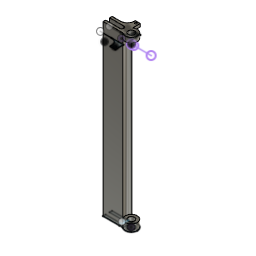
Aft_Flap (Autodesk Fusion 360 design; units mm, degrees)
Autodesk Fusion 360 part; units mm, degrees
note: some values were not read from the file. Set by a fixed rule: which sketch regions a step uses.
sketch "Sketch1" plane through (0, 0, 0) normal (0, 0, 1) x (1, 0, 0)
  circle A0 centre (0, 0) radius 3.2
  circle A1 centre (0, 0) radius 6
  line L0 (-7.5, -4.5) -> (-3.9686, -4.5)
  line L1 (-3.9686, -4.5) -> (-3.9686, 4.5)
  line L2 (-3.9686, 4.5) -> (-7.5, 4.5)
  line L3 (-7.5, 0) -> (-7.5, 0)
  line L4 (-7.5, 4.5) -> (-23.9686, 4.5)
  line L5 (-23.9686, 4.5) -> (-23.9686, 2)
  line L6 (-23.9686, 2) -> (-9.5, 2)
  line L7 (-7.5, 2) -> (-7.5, 4.5)
  line L8 (-7.5, -4.5) -> (-23.9686, -4.5)
  line L9 (-23.9686, -4.5) -> (-23.9686, -2)
  line L10 (-23.9686, -2) -> (-9.5, -2)
  line L11 (-7.5, -2) -> (-7.5, -4.5)
  arc A2 (-7.5, 0) -> (-9.5, 2) centre (-9.5, 0) ccw
  arc A3 (-9.5, -2) -> (-7.5, 0) centre (-9.5, 0) ccw
  dimension "d1" = 6.4
  dimension "d2" = 12
  dimension "d10" = 2
  dimension "d11" = 2
  dimension "d12" = 7.5
  dimension "d15" = 9
  dimension "d16" = 2
  dimension "d17" = 2
  dimension "d19" = 2.5
  dimension "d32" = 2.5
  dimension "d33" = 20
  dimension "d34" = 20
  constraint coincident A0.centre A1.centre
  constraint horizontal L2
  constraint coincident A1 L1.end
  constraint horizontal L4
  constraint vertical L5
  constraint horizontal L6
  constraint vertical L7
  constraint horizontal L8
  constraint vertical L9
  constraint horizontal L10
  constraint vertical L11
  constraint coincident L7.start L6
  constraint tangent L6 A2
  constraint coincident L0.start L3
  constraint coincident L11.start L10
  constraint tangent L10 A3
  constraint parallel L0 L8
  constraint coincident L1 L0.end
  constraint coincident L0.end L1.start
  constraint perpendicular L0 L1
  measures "d1" diameter of A0
  measures "d2" diameter of A1
  measures "d10" distance of A0.centre L10
  measures "d11" distance of A0.centre L6
  measures "d12" distance of A0.centre L11
  measures "d15" distance of L0.end L1.end
  measures "d16" radius of A2
  measures "d17" radius of A3
  measures "d19" distance of L4 L6
  measures "d32" distance of L8 L10
  measures "d33" distance of L1 L5
  measures "d34" distance of L1 L9
extrude "Extrude1" add sketch "Sketch1" along normal blind 7 contours A1 L1 | A1 L1 makes body 1
extrude "Extrude2" add sketch "Sketch1" along normal blind 5 from surface at 165 separate body contours A1 L1 | A1 L1 makes body 2
extrude "Extrude3" add sketch "Sketch1" along normal blind 170 contours A1 L0 L2 L4 L5 L6 L8 L9 L10 A2 A3 bodies 1 2
ref_plane "WorkPlane1" through (-7.8276, 0, 160) normal (0, 0, 1) x (1, 0, 0)
sketch "Sketch2" plane through (-9.7903, 0, 160) normal (0, 0, 1) x (1, 0, 0)
  line L0 (6.2903, -4.5) -> (1.2903, -4.5)
  line L1 (1.2903, -11.5) -> (1.2903, -12.5)
  line L2 (1.2903, -12.5) -> (6.2903, -12.5)
  line L3 (6.2903, -12.5) -> (6.2903, -4.5)
  circle A0 centre (3.7903, -10.5) radius 1
  line L4 (-5.7097, -4.5) -> (-16.9277, -4.5)
  arc A1 (1.2903, -11.5) -> (-5.7097, -4.5) centre (-5.7097, -11.5) ccw
  line L5 (1.2903, -4.5) -> (-5.7097, -4.5)
  line L6 (29.7903, 0) -> (12.2903, 0)
  line L7 (6.2903, 12.5) -> (6.2903, 4.5)
  line L8 (6.2903, 4.5) -> (1.2903, 4.5)
  circle A2 centre (3.7903, 10.5) radius 1
  arc A3 (-5.7097, 4.5) -> (1.2903, 11.5) centre (-5.7097, 11.5) ccw
  line L9 (1.2903, 4.5) -> (-5.7097, 4.5)
  line L10 (-5.7097, 4.5) -> (-16.9277, 4.5)
  line L11 (1.2903, 12.5) -> (6.2903, 12.5)
  line L12 (1.2903, 11.5) -> (1.2903, 12.5)
  point P0 (9.7903, 0)
  point P1 (9.7903, 0)
  dimension "d21" = 4.5
  dimension "d22" = 5
  dimension "d23" = 3.5
  dimension "d24" = 8
  dimension "d25" = 2
  dimension "d26" = 6
  dimension "d27" = 2.5
  dimension "d31" = 7
  constraint horizontal L0
  constraint vertical L1
  constraint horizontal L2
  constraint vertical L3
  constraint perpendicular L1 L4
  constraint coincident L0.end L1
  constraint coincident L0.end L4
  constraint tangent L1 A1
  constraint tangent L4 A1
  constraint symmetric L0.start L6 L7.end
  constraint symmetric L0.end L6 L8.end
  constraint symmetric L1.end L6 L11.start
  constraint symmetric L2.end L6 L7.start
  constraint symmetric A0 L6 A2
  constraint symmetric P1 L6 P0
  constraint symmetric L4.end L6 L10.end
  constraint symmetric L1.start L6 A3.end
  constraint symmetric L4.start L6 A3.start
  constraint symmetric A1 L6 A3
  measures "d21" distance of L0 P1
  measures "d22" distance of L1 L3
  measures "d23" distance of L3 P1
  measures "d24" distance of L0 L2
  measures "d25" diameter of A0
  measures "d26" distance of L0 A0.centre
  measures "d27" distance of L3 A0.centre
  measures "d31" radius of A1
extrude "Extrude4" add sketch "Sketch2" along normal up to surface (3 mm away) from surface at 7 contours L7 L8 A3 L9 L11 L12 bodies 1
